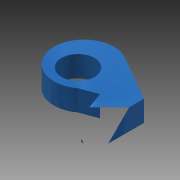
# Autodesk Inventor part: OfflineExtruderTensionCam
Saved by Autodesk Inventor 2015 SP1 (Build 190203100, 203)
## iProperties
Created: 2015-05-04
Part Number: OfflineExtruderTensionCam
Material: ABS Plastic
Document SubType Name: Modeling
Designer: Jack
Density: 1.06 g/cm^3
Appearance: Cyan
Author: Jack
Autodesk Inventor part; units mm, degrees
ref_plane "YZ Plane" through (0, 0, 0) normal (1, 0, 0) x (0, 1, 0)
ref_plane "XZ Plane" through (0, 0, 0) normal (0, 1, 0) x (-1, 0, 0)
ref_plane "XY Plane" through (0, 0, 0) normal (0, 0, 1) x (1, 0, 0)
sketch "Sketch1" plane through (0, 0, 0) normal (0, 0, 1) x (1, 0, 0)
  arc A0 (5, 8.6603) -> (6, -8) centre (0, 0) ccw
  line L0 (5, 8.6603) -> (20, 0)
  line L1 (20, 0) -> (20, -16)
  line L2 (20, -16) -> (15, -16)
  line L3 (15, -16) -> (11.3603, -6)
  line L4 (11.3603, -6) -> (6, -8)
  dimension "d0" = 20
  dimension "d4" = 5
  dimension "d5" = 10
  dimension "d6" = 16
  dimension "d7" = 15
  dimension "d8" = 120
  dimension "d9" = 110
  dimension "d20" = 8
  constraints: 10 end point, 2 point on circle, 1 centre point, 1 coincident, 1 horizontal alignment, 1 perpendicular, 1 tangent
  measures "d0" diameter of A0
  measures "d4" distance of L1.end L2.end
  measures "d5" vertical distance of L2.end L3.end
  measures "d6" distance of L0.end L1.end
  measures "d7" horizontal distance of L0.start L0.end
  measures "d8" angle of L0 L1
  measures "d9" angle of L2 L3
  measures "d20" vertical distance of point (0, 0) L4.end
extrude "Extrusion1" add sketch "Sketch1" along normal blind 7
sketch "Sketch2" plane through (0, 0, 7) normal (0, 0, 1) x (1, 0, 0)
  arc A0 (5, 8.6603) -> (6, -8) centre (0, 0) ccw projected
  point P0 (0, -2)
  dimension "d12" = 2
  constraints: 1 vertical alignment
  measures "d12" distance of A0.centre point (0, -2)
hole "Hole1" at (0, -2, 7) direction (0, 0, -1) diameter 11 depth 8 tip angle 118
body "Solid1"
